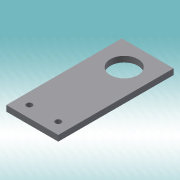
# Autodesk Inventor part: 回転軸取り付け板
Saved by Autodesk Inventor 2015 (Build 190159000, 159)
## iProperties
Created: 2016-03-21
Part Number: 回転軸取り付け板
Material: 一般
Document SubType Name: Modeling
Designer: buzztaka
Density: 1 g/cm^3
Appearance: 既定
Author: buzztaka
Autodesk Inventor part; units mm, degrees
ref_plane "YZ Plane" through (0, 0, 0) normal (1, 0, 0) x (0, 1, 0)
ref_plane "XZ Plane" through (0, 0, 0) normal (0, 1, 0) x (-1, 0, 0)
ref_plane "XY Plane" through (0, 0, 0) normal (0, 0, 1) x (1, 0, 0)
sketch "スケッチ1" plane through (0, 0, 0) normal (0, 0, 1) x (1, 0, 0)
  line L0 (0, 0) -> (45, 0)
  line L1 (45, 0) -> (45, 100)
  line L2 (45, 100) -> (0, 100)
  line L3 (0, 100) -> (0, 0)
  dimension "d0" = 100
  dimension "d1" = 45
  constraints: 8 end point, 2 parallel, 1 horizontal, 1 perpendicular
  measures "d0" distance of L2.end L0.start
  measures "d1" distance of L0.start L0.end
extrude "押し出し1" add sketch "スケッチ1" along normal blind 5
sketch "スケッチ2" plane through (0, 0, 5) normal (0, 0, 1) x (1, 0, 0)
  line L0 (0, 0) -> (45, 0) projected
  point P0 (22.6447, 79.5)
  dimension "d4" = 79.5
  measures "d4" distance from line of L0 point (22.645, 79.5)
hole "穴1" at (22.6447, 79.5, 5) direction (0, 0, -1) diameter 24 end through all
sketch "スケッチ3" plane through (0, 0, 0) normal (0, 0, -1) x (-1, 0, 0)
  line L0 (0, 0) -> (-45, 0) projected
  line L1 (-45, 0) -> (-45, 100) projected
  line L2 (0, 100) -> (0, 0) projected
  point P0 (-10, 10)
  point P1 (-35, 10)
  dimension "d12" = 10
  dimension "d13" = 10
  dimension "d14" = 10
  dimension "d15" = 10
  measures "d12" distance from line of point (-10, 10) L0
  measures "d13" distance from line of L0 point (-35, 10)
  measures "d14" distance from line of L1 point (-35, 10)
  measures "d15" distance from line of point (-10, 10) L2
hole "穴2" at (10, 10, 0) at (35, 10, 0) direction (0, 0, 1) diameter 5 end through all
